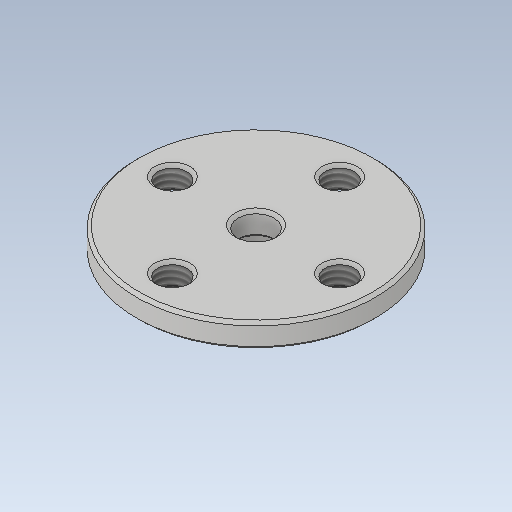
# Autodesk Inventor part: motortarcsa
Saved by Autodesk Inventor 2020 (Build 240168000, 168)
## iProperties
Created: 2013-06-07
Part Number: motortarcsa
Material: Generic
Document SubType Name: Modeling
Designer: Horváth Patrik
Density: 1 g/cm^3
Appearance: Default
Author: Horváth Patrik
Revision Number: ANY
Autodesk Inventor part; units mm, degrees
ref_plane "YZ Plane" through (0, 0, 0) normal (1, 0, 0) x (0, 1, 0)
ref_plane "XZ Plane" through (0, 0, 0) normal (0, 1, 0) x (-1, 0, 0)
ref_plane "XY Plane" through (0, 0, 0) normal (0, 0, 1) x (1, 0, 0)
sketch "Sketch1" plane through (0, 0, 0) normal (0, 0, 1) x (1, 0, 0)
  line L0 (-12, 0) -> (2, 0) construction
  line L1 (0, -5.4) -> (0, 0.9) construction
  line L2 (-1.5, 0) -> (-10, 0)
  line L3 (-10, 0) -> (-10, -2)
  line L4 (-10, -2) -> (-4.5, -2)
  line L5 (-4.5, -2) -> (-4.5, -4.5)
  line L6 (-4.5, -4.5) -> (-3, -4.5)
  line L7 (-3, -4.5) -> (-3, -2)
  line L8 (-3, -2) -> (-1.5, -2)
  line L9 (-1.5, 0) -> (-1.5, -2)
  point P0 (0, 0)
  dimension "d0" = 1.5
  dimension "d1" = 3
  dimension "d2" = 4.5
  dimension "d3" = 10
  dimension "d4" = 2
  dimension "d5" = 4.5
  constraints: 16 end point, 6 perpendicular, 2 collinear, 1 point on line, 1 vertical
  measures "d0" distance between parallel lines of L1 L9
  measures "d1" distance between parallel lines of L1 L7
  measures "d2" distance between parallel lines of L1 L5
  measures "d3" distance between parallel lines of L1 L3
  measures "d4" distance between parallel lines of L0 L4
  measures "d5" distance between parallel lines of L0 L6
revolve "Revolution1" add sketch "Sketch1" angle 360 about axis through (0, -10, 0) along (0, 1, 0)
sketch "Sketch2" plane through (0, 0, 0) normal (0, 1, 0) x (1, 0, 0)
  line L0 (-14, 0) -> (14, 0) construction
  line L1 (0, 14) -> (0, -14) construction
  point P0 (0, 0)
  point P1 (0, 7)
  point P2 (0, -7)
  point P3 (-7, 0)
  point P4 (7, 0)
  dimension "d7" = 14
  dimension "d8" = 14
  constraints: 4 point on line, 2 symmetric about line
  measures "d7" distance of point (0, 7) point (0, -7)
  measures "d8" distance of point (7, 0) point (-7, 0)
hole "Hole1" at (0, 0, -7) at (0, 0, 7) at (-7, 0, 0) at (7, 0, 0) direction (0, -1, 0) diameter 2.459 depth 8.8 thread size "M3x0.5" class "6H" standard "ISO Metric profile"
chamfer "Chamfer1" distance 0.25 angle 45 16 edges at (10, 0, 0) (10, -2, 0) (0, 0, -8.2295) (7, 0, -1.2295) (-7, 0, -1.2295) (0, 0, 5.7705) (4.5, -2, 0) (4.5, -4.5, 0) (3, -4.5, 0) (3, -2, 0) (1.5, -2, 0) (1.5, 0, 0) (0, -2, -8.2295) (7, -2, -1.2295) (-7, -2, -1.2295) (0, -2, 5.7705)
body "Solid2"
